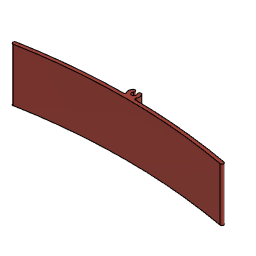
Catcher Mount v1 (Autodesk Fusion 360 design; units mm, degrees)
Autodesk Fusion 360 part; units mm, degrees
note: some values were not read from the file. Chosen so that the rebuilt part matches the saved one: which face or edge a step refers to. Set by a fixed rule: which sketch regions a step uses.
sketch "Sketch1" plane through (0, 0, 0) normal (0, 0, 1) x (1, 0, 0)
  arc A0 (-0.6128, 3.3142) -> (0.6128, 3.3142) centre (0, 2.8) ccw
  line L0 (0, 2.8) -> (-0.6128, 3.3142) construction
  line L1 (0, 2.8) -> (0.6128, 3.3142) construction
  line L2 (0, 0) -> (0, 2.8)
  arc A1 (0.9287, 4.5713) -> (0.6128, 3.3142) centre (1.2257, 3.8285) ccw
  line L3 (0, 2.8) -> (0.9167, 2.8) construction
  arc A2 (-0.6128, 3.3142) -> (-0.9287, 4.5713) centre (-1.2257, 3.8285) ccw
  circle A3 centre (0, 2.8) radius 2
  arc A4 (37.5, -3.4902) -> (-37.5, -3.4902) centre (0, -203.2) ccw
  line L4 (-1.7264, 0.8) -> (1.5124, 0.8) construction
  arc A5 (37.7215, -2.3108) -> (-37.7215, -2.3108) centre (0, -203.2) ccw
  line L5 (-37.7215, -2.3108) -> (-37.5, -3.4902)
  line L6 (37.5, -3.4902) -> (37.7215, -2.3108)
  dimension "d1" = 0.8
  dimension "d4" = 0.8
  dimension "d5" = 40
  dimension "d7" = 2
  dimension "d9" = 203.2
  dimension "d10" = 75
  dimension "d11" = 0.8
  dimension "d12" = 1.2
  constraint coincident L2.start origin
  constraint coincident A0.centre L0.start
  constraint vertical L2
  constraint symmetric A0.start A0.end L2
  constraint perpendicular L2 L3
  constraint tangent A0 A1
  constraint symmetric A0.end L2 A0.start
  constraint symmetric L2 A1.start A2.end
  constraint symmetric L2 A1 A2
  constraint concentric A0 A3
  constraint coincident A1.start A3
  constraint vertical L2.start A4.centre
  constraint coincident L2.start A4
  constraint symmetric L2 A4.start A4.end
  constraint horizontal L4
  constraint tangent A3 L4
  measures "d1" radius of A0
  measures "d4" radius of A1
  measures "d5" angle of L1 L3
  measures "d7" radius of A3
  measures "d9" radius of A4
  measures "d10" distance of A4.start A4.end
  measures "d11" distance of L2.start L4
extrude "Extrude1" add sketch "Sketch1" along normal blind 19 contours A0 L2 A2 A3 A5 | A0 L2 A1 A3 A5 | L2 A3 A5 | L2 A3 A5 | L2 A3 A4 A5 L5 | L2 A3 A4 A5 L6
extrude "Extrude2" add sketch "Sketch1" along normal blind 1 contours A0 A1 A2 A3
fillet "Fillet1" radius 0.6 2 edges at (0.9287, 4.5713, 10) (-0.9287, 4.5713, 10)
fillet "Fillet2" radius 0.6 2 edges at (37.7215, -2.3108, 9.5) (37.5, -3.4902, 9.5)
fillet "Fillet2" radius 0.6 2 edges at (-37.5, -3.4902, 9.5) (-37.7215, -2.3108, 9.5)
fillet "Fillet3" radius 0.4 2 edges at (1.1953, 1.1965, 9.5) (-1.1953, 1.1965, 9.5)
equation "d1 = ( 1.6 / 2 ) * 1 mm"
equation "d4 = d1"
equation "d7 = d1 + 1.2 mm"
